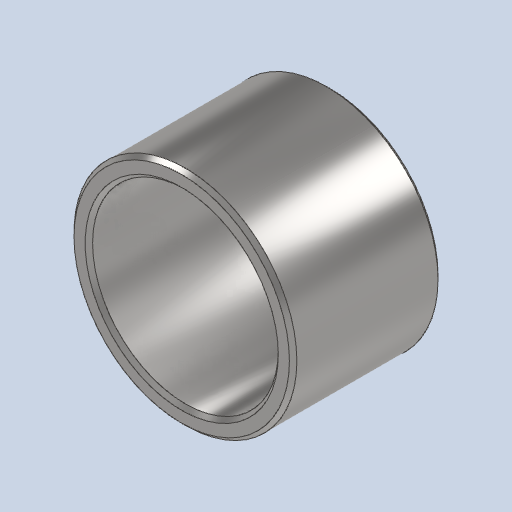
# Autodesk Inventor part: WSSS-12-10-8
Saved by Autodesk Inventor 2022 (Build 260153000, 153)
## iProperties
Part Number: WSSS-12-10-8
Material: ステンレス鋼 AISI 304
Document SubType Name: Modeling
Designer: Masato Kubotera
Density: 6.75934 g/cm^3
Appearance: 半つや出し
Catalog Web Link: https://jp.misumi-ec.com/vona2/detail/110302677010/?HissuCode=WSSS12-10-8
Description: ReadyMade
Mass: 1.85 g
Surface Area: 6.05841 cm^2
Volume: 0.273696 cm^3
Author: Masato Kubotera
Autodesk Inventor part; units mm, degrees
ref_plane "YZ Plane" through (0, 0, 0) normal (1, 0, 0) x (0, 1, 0)
ref_plane "XZ Plane" through (0, 0, 0) normal (0, 1, 0) x (-1, 0, 0)
ref_plane "XY Plane" through (0, 0, 0) normal (0, 0, 1) x (1, 0, 0)
sketch "スケッチ1" plane through (0, 0, 0) normal (0, 1, 0) x (-1, 0, 0)
  line L0 (-5.2, 8) -> (-5.8, 8)
  line L1 (-6, 7.8) -> (-6, 0.2)
  line L2 (-5.8, 0) -> (-5.2, 0)
  line L3 (-5, 0.2) -> (-5, 7.8)
  line L4 (-5, 8) -> (-6, 0) construction
  line L5 (-6, 8) -> (-5, 0) construction
  line L6 (0, -1.6) -> (0, 9.6) projected
  line L7 (-5.8, 8) -> (-6, 7.8)
  line L8 (-6, 0.2) -> (-5.8, 0)
  line L9 (-5.2, 0) -> (-5, 0.2)
  line L10 (-5, 7.8) -> (-5.2, 8)
  point P0 (0, 0)
  point P1 (-5.5, 4)
  dimension "d0" = 10
  dimension "d1" = 12
  dimension "d2" = 8
  dimension "d3" = 0.2
  dimension "d4" = 0.2
  dimension "d5" = 0.2
  dimension "d6" = 0.2
  dimension "d7" = 0.2
  dimension "d8" = 0.2
  dimension "d9" = 0.2
  dimension "d10" = 0.2
  constraints: 20 end point, 9 point on line, 2 midpoint, 2 parallel, 1 horizontal, 1 perpendicular
  measures "d0" diameter of L3 L6
  measures "d1" diameter of L5.start L6
  measures "d2" distance of L5.start L4.end
  measures "d3" distance of L0.end L5.start
  measures "d4" distance of L1.start L5.start
  measures "d5" distance of L1.end L4.end
  measures "d6" distance of L2.start L4.end
  measures "d7" distance of L2.end L5.end
  measures "d8" distance of L3.start L5.end
  measures "d9" distance of L3.end L4.start
  measures "d10" distance of L0.start L4.start
revolve "回転1" add sketch "スケッチ1" angle 360 about axis through (0, 0, -10) along (0, 0, 1)
equation "\"d4\" = d3"
equation "\"d5\" = d3"
equation "\"d6\" = d5"
equation "\"d7\" = d3"
equation "\"d8\" = d7"
equation "\"d9\" = d3"
equation "\"d10\" = d9"
